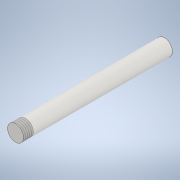
# Autodesk Inventor part: Eje roscado base soporte tubo
Saved by Autodesk Inventor 2021 (Build 250183000, 183)
## iProperties
Created: 2021-05-02
Part Number: Eje roscado base soporte tubo
Material: Steel AISI 1020 107 HR
Document SubType Name: Modeling
Designer: maaro
Density: 7.87 g/cm^3
Appearance: Steel
Author: maaro
Autodesk Inventor part; units mm, degrees
ref_plane "YZ Plane" through (0, 0, 0) normal (1, 0, 0) x (0, 1, 0)
ref_plane "XZ Plane" through (0, 0, 0) normal (0, 1, 0) x (-1, 0, 0)
ref_plane "Work Plane1" through (0, 0, 20) normal (0, 0, 1) x (1, 0, 0)
sketch "Sketch1" plane through (0, 0, 20) normal (0, 0, 1) x (1, 0, 0)
  circle A0 centre (-20, -75) radius 8 projected
  point P0 (0, 0)
extrude "Extrusion1" add sketch "Sketch1" against normal blind 147.993
thread "Thread2" size "M16x2" class "6g" standard "ANSI Metric M Profile" length 10
body "Solid1"
